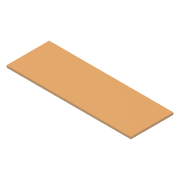
# Autodesk Inventor part: AcrylicLogo
Saved by Autodesk Inventor 2014 (Build 180170000, 170)
## iProperties
Created: 2014-08-11
Part Number: AcrylicLogo
Material: Generic
Document SubType Name: Modeling
Designer: Peele
Density: 1 g/cm^3
Appearance: Clear - Yellow
Author: Peele
Autodesk Inventor part; units mm, degrees
ref_plane "YZ Plane" through (0, 0, 0) normal (1, 0, 0) x (0, 1, 0)
ref_plane "XZ Plane" through (0, 0, 0) normal (0, 1, 0) x (-1, 0, 0)
ref_plane "XY Plane" through (0, 0, 0) normal (0, 0, 1) x (1, 0, 0)
sketch "Sketch1" plane through (0, 0, 0) normal (0, 0, 1) x (1, 0, 0)
  line L0 (-87.5, -30) -> (87.5, -30)
  line L1 (87.5, -30) -> (87.5, 30)
  line L2 (87.5, 30) -> (-87.5, 30)
  line L3 (-87.5, 30) -> (-87.5, -30)
  line L4 (-87.5, -30) -> (87.5, 30) construction
  line L5 (87.5, -30) -> (-87.5, 30) construction
  point P0 (0, 0)
  dimension "d0" = 60
  dimension "d1" = 175
  constraints: 12 end point, 2 midpoint, 2 parallel, 1 horizontal, 1 perpendicular
  measures "d0" distance of L2.end L0.start
  measures "d1" distance of L0.start L0.end
extrude "Extrusion1" add sketch "Sketch1" along normal blind 3
body "Solid1"
